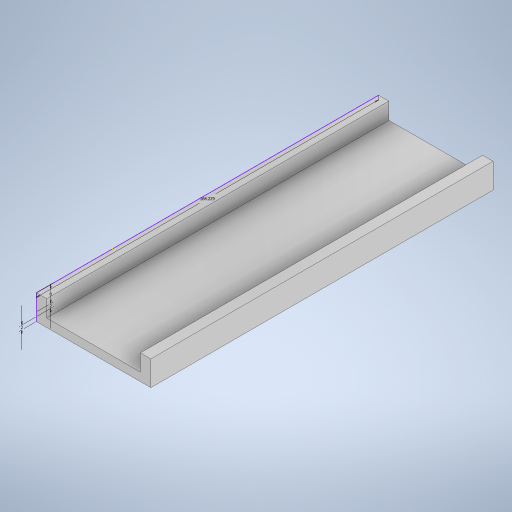
# Autodesk Inventor part: Flange
Saved by Autodesk Inventor 2024 (Build 280153000, 153)
## iProperties
Created: 2023-12-18
Part Number: Flange
Material: Aluminum 6061-AHC
Document SubType Name: Modeling
Designer: pratikhya
Density: 2.7 g/cm^3
Appearance: Aluminum - Dark
Author: pratikhya
Autodesk Inventor part; units mm, degrees
ref_plane "YZ Plane" through (0, 0, 0) normal (1, 0, 0) x (0, 1, 0)
ref_plane "XZ Plane" through (0, 0, 0) normal (0, 1, 0) x (-1, 0, 0)
ref_plane "XY Plane" through (0, 0, 0) normal (0, 0, 1) x (1, 0, 0)
sketch "Sketch1" plane through (0, 0, 0) normal (1, 0, 0) x (0, 1, 0)
  line L0 (0, 36.5286) -> (0, -127.7004)
  line L1 (0, 36.5286) -> (-8, 36.5286)
  line L2 (-8, 36.5286) -> (-8, -127.7004)
  line L3 (-8, -127.7004) -> (-5.4683, -127.7004)
  line L4 (-5.4683, -127.7004) -> (-2.7019, -127.7004)
  line L5 (-2.7019, -127.7004) -> (0, -127.7004)
  line L6 (-8, 36.5286) -> (-10, 36.5286)
  line L7 (-10, 36.5286) -> (-12, 36.5286)
  line L8 (-12, 36.5286) -> (-12, -127.7004)
  line L9 (-12, -127.7004) -> (-8, -127.7004)
  point P0 (0, 0)
  dimension "d0" = 164.229
  dimension "d1" = 8
  dimension "d2" = 2
  dimension "d3" = 2
  constraints: 20 end point, 3 perpendicular, 2 horizontal, 2 point on line, 1 collinear, 1 vertical
  measures "d0" distance of L0.start L0.end
  measures "d1" distance of L0.start L1.end
  measures "d2" distance of L1.end L6.end
  measures "d3" distance of L6.end L7.end
extrude "Extrusion1" add sketch "Sketch1" along normal blind 5 contours L0 L5 L4 L3 L2 L1
sketch "Sketch2" plane through (0, 0, 0) normal (-1, 0, 0) x (0, 0, 1)
  point P0 (0, 0)
extrude "Extrusion2" add sketch "Sketch1" along normal blind 50 contours L2 L9 L8 L7 L6
sketch "Sketch3" plane through (50, 0, 0) normal (1, 0, 0) x (0, 0, -1)
  line L0 (-36.5286, -12) -> (127.7004, -12) projected
  line L1 (-36.5286, 0) -> (-36.5286, -12) projected
  line L2 (-36.5286, -12) -> (-36.5286, 0)
  line L3 (127.7004, -12) -> (127.7004, 0) projected
  line L4 (-36.5286, 0) -> (127.7004, 0)
  line L5 (127.7004, 0) -> (127.7004, -12)
  line L6 (127.7004, -12) -> (-36.5286, -12)
  point P0 (0, 0)
  dimension "d8" = 12
  constraints: 8 end point, 2 collinear, 1 horizontal, 1 perpendicular
  measures "d8" distance of L0.start L1.start
extrude "Extrusion3" add sketch "Sketch3" along normal blind 5
body "Solid1"
